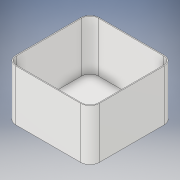
# Autodesk Inventor part: case_bottom
Saved by Autodesk Inventor 2019 (Build 230136000, 136)
## iProperties
Created: 2019-01-23
Part Number: case_bottom
Material: Generic
Document SubType Name: Modeling
Designer: jmc
Density: 1 g/cm^3
Appearance: PET White
Author: jmc
Autodesk Inventor part; units mm, degrees
ref_plane "YZ Plane" through (0, 0, 0) normal (1, 0, 0) x (0, 1, 0)
ref_plane "XZ Plane" through (0, 0, 0) normal (0, 1, 0) x (-1, 0, 0)
ref_plane "XY Plane" through (0, 0, 0) normal (0, 0, 1) x (1, 0, 0)
sketch "Sketch1" plane through (0, 0, 0) normal (0, 1, 0) x (-1, 0, 0)
  line L0 (90, 70) -> (90, -70)
  arc A0 (70, -90) -> (90, -70) centre (70, -70) ccw
  line L1 (70, -90) -> (-70, -90)
  arc A1 (-90, -70) -> (-70, -90) centre (-70, -70) ccw
  line L2 (-90, -70) -> (-90, 70)
  arc A2 (-70, 90) -> (-90, 70) centre (-70, 70) ccw
  line L3 (-70, 90) -> (70, 90)
  arc A3 (90, 70) -> (70, 90) centre (70, 70) ccw
  line L4 (-90, 90) -> (90, -90)
  line L5 (90, 90) -> (-90, -90)
  line L6 (0, 101.9126) -> (0, -124.7005)
  line L7 (136.9186, 0) -> (-105.9116, 0)
  point P0 (0, 0)
  constraints: 16 end point, 8 point on circle, 8 tangent, 4 centre point, 4 perpendicular, 3 equal radius, 2 parallel
extrude "Extrusion1" add sketch "Sketch1" along normal blind 110
shell "Shell1" thickness 2 removed faces 1 at (23.3333, 110, 30)
body "Solid1"
